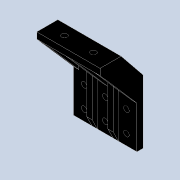
# Autodesk Inventor part: X Axis Drag Chain Support Mount
Saved by Autodesk Inventor 2022 (Build 260153000, 153)
## iProperties
Created: 2021-10-30
Part Number: X Axis Drag Chain Support Mount
Material: Generic
Document SubType Name: Modeling
Designer: Coy
Density: 1 g/cm^3
Appearance: Anodized - Black
Author: Coy
Autodesk Inventor part; units mm, degrees
ref_plane "YZ Plane" through (0, 0, 0) normal (1, 0, 0) x (0, 1, 0)
ref_plane "XZ Plane" through (0, 0, 0) normal (0, 1, 0) x (-1, 0, 0)
sketch "Sketch1" plane through (0, 0, 0) normal (0, 0, 1) x (1, 0, 0)
  line L0 (0, 0) -> (-60, 0)
  line L1 (-60, 0) -> (-60, 60)
  line L2 (-60, 60) -> (0, 60)
  line L3 (0, 60) -> (0, 0)
  dimension "d0" = 60
  dimension "d1" = 60
  constraints: 8 end point, 2 parallel, 1 horizontal, 1 perpendicular
  measures "d0" distance of L1.end L2.end
  measures "d1" distance of L0.end L1.end
extrude "Extrusion1" add sketch "Sketch1" along normal blind 6
sketch "Sketch2" plane through (0, 0, 6) normal (0, 0, 1) x (1, 0, 0)
  line L0 (0, 60) -> (-60, 60) projected
  line L1 (-60, 60) -> (-60, 0) projected
  line L2 (0, 60) -> (-60, 60)
  line L3 (-60, 60) -> (-60, 40)
  line L4 (-60, 40) -> (0, 40)
  line L5 (0, 40) -> (0, 60)
  line L6 (-60, 0) -> (0, 0) construction
  line L7 (-30, 0) -> (-30, 40) construction
  line L8 (-30, 20) -> (-30, 40) construction
  line L9 (-30, 20) -> (-30, 0) construction
  line L10 (-60, 30) -> (0, 30) construction
  line L11 (0, 0) -> (0, 60) construction
  line L12 (-60, 10) -> (0, 10) construction
  circle A0 centre (-50, 30) radius 2.6
  circle A1 centre (-30, 30) radius 2.6
  circle A2 centre (-10, 30) radius 2.6
  circle A3 centre (-50, 10) radius 2.6
  circle A4 centre (-30, 10) radius 2.6
  circle A5 centre (-10, 10) radius 2.6
  dimension "d4" = 20
  dimension "d5" = 5.2
  dimension "d6" = 5.2
  dimension "d7" = 5.2
  dimension "d8" = 5.2
  dimension "d9" = 5.2
  dimension "d10" = 5.2
  dimension "d11" = 20
  dimension "d12" = 20
  dimension "d13" = 20
  dimension "d14" = 20
  dimension "d15" = 20
  constraints: 18 end point, 8 midpoint, 6 centre point, 6 point on line, 2 collinear, 2 parallel, 2 perpendicular, 1 horizontal
  measures "d4" distance of L3.end L2.end
  measures "d5" diameter of A0
  measures "d6" diameter of A1
  measures "d7" diameter of A2
  measures "d8" diameter of A3
  measures "d9" diameter of A4
  measures "d10" diameter of A5
  measures "d11" distance of A1.centre A0.centre
  measures "d12" distance of A4.centre A3.centre
  measures "d13" distance of A1.centre A2.centre
  measures "d14" distance of A4.centre A5.centre
  measures "d15" distance between parallel lines of L10 L12
extrude "Extrusion2" cut sketch "Sketch2" against normal up to next contours A0 | A1 | A2 | A3 | A4 | A5
sketch "Sketch3" plane through (0, 0, 0) normal (1, 0, 0) x (0, 0, -1)
  line L0 (0, 60) -> (0, 0) construction
  line L1 (0, 0) -> (0, 135.0487) construction
  line L2 (-21, 0) -> (-21, 135.0487) construction
  line L3 (-21, 86) -> (-41, 86)
  line L4 (-41, 86) -> (-41, 80)
  line L5 (-41, 80) -> (-21, 80)
  line L6 (-21, 80) -> (-21, 86)
  line L7 (0, 60) -> (-6, 60) projected
  line L8 (0, 60) -> (-6, 60) projected
  line L9 (-21, 86) -> (0, 60)
  line L10 (-6, 60) -> (-6, 0) projected
  line L11 (-6, 60) -> (-21, 80)
  dimension "d18" = 21
  dimension "d19" = 20
  dimension "d20" = 6
  dimension "d21" = 20
  constraints: 16 end point, 2 parallel, 2 vertical, 1 horizontal, 1 perpendicular, 1 point on line
  measures "d18" distance between parallel lines of L1 L2
  measures "d19" distance of L5.end L4.end
  measures "d20" distance of L4.end L3.end
  measures "d21" distance between parallel lines of L7 L5
extrude "Extrusion3" add sketch "Sketch3" against normal up to surface (60 mm away)
sketch "Sketch4" plane through (0, 80, 41) normal (0, 0, 1) x (1, 0, 0)
  line L0 (0, 0) -> (-60, 0) projected
  line L1 (0, 0) -> (-5, 0)
  line L2 (-5, 0) -> (-5, -40)
  line L3 (-5, -40) -> (0, -40)
  line L4 (0, -40) -> (0, 0)
  circle A0 centre (-10, -50) radius 2.6 projected
  line L5 (-32.5, 0) -> (-32.5, -40)
  line L6 (-27.5, 0) -> (-32.5, 0)
  line L7 (-27.5, -40) -> (-27.5, 0)
  line L8 (-32.5, -40) -> (-27.5, -40)
  line L9 (-60, 0) -> (-60, -40)
  line L10 (-55, 0) -> (-60, 0)
  line L11 (-55, -40) -> (-55, 0)
  line L12 (-60, -40) -> (-55, -40)
  point P0 (0, -80)
  dimension "d24" = 5
  dimension "d25" = 10
  dimension "d28" = 27.5
  constraints: 24 end point, 2 horizontal, 2 parallel, 1 perpendicular, 16 other
  measures "d24" distance of L3.end L2.end
  measures "d25" distance from line of A0.centre L3
  measures "d28" distance of L1.end L5.start
extrude "Extrusion4" add sketch "Sketch4" against normal up to next contours L4 L3 L2 L0 | L11 L12 L9 L0 | L7 L8 L5 L0
chamfer "Chamfer1" distance 40 distance2 35 1 edges at (-2.5, 40, 41) measured on face at (-30.8333, 84, 41)
chamfer "Chamfer2" distance 40 distance2 35 1 edges at (-30, 40, 41) measured on face at (-30.8333, 84, 41)
chamfer "Chamfer3" distance 40 distance2 35 1 edges at (-57.5, 40, 41) measured on face at (-30.8333, 84, 41)
sketch "Sketch5" plane through (-55, 80, 21) normal (0, -1, 0) x (1, 0, 0)
  line L0 (-5, 0) -> (-5, 20) construction
  line L1 (-5, 10) -> (55, 10) construction
  line L2 (55, -15) -> (55, 20) construction
  circle A0 centre (11.25, 10) radius 2.6
  circle A1 centre (38.75, 10) radius 2.6
  line L3 (0, 20) -> (0, 0) projected
  line L4 (27.5, 20) -> (27.5, 0) projected
  point P0 (55, -21)
  dimension "d44" = 5.2
  dimension "d45" = 5.2
  dimension "d46" = 11.25
  dimension "d47" = 11.25
  constraints: 3 point on line, 2 centre point, 2 end point, 1 horizontal, 1 midpoint
  measures "d44" diameter of A0
  measures "d45" diameter of A1
  measures "d46" distance from line of L3 A0.centre
  measures "d47" distance from line of L4 A1.centre
extrude "Extrusion5" cut sketch "Sketch5" against normal up to next
ref_plane "Work Plane1" through (0, 0, 11) normal (0, 0, 1) x (1, 0, 0)
sketch "Sketch7" plane through (0, 0, 11) normal (0, 0, 1) x (1, 0, 0)
  line L0 (-60, 0) -> (0, 0) projected
  line L1 (-17.5, 0) -> (-22.5, 0)
  line L2 (-22.5, 0) -> (-22.5, 70)
  line L3 (-22.5, 70) -> (-17.5, 70)
  line L4 (-17.5, 70) -> (-17.5, 0)
  circle A0 centre (-10, 30) radius 2.6 projected
  line L5 (-30, 0) -> (-30, 54.0913) construction
  line L6 (-42.5, 0) -> (-37.5, 0)
  line L7 (-37.5, 0) -> (-37.5, 70)
  line L8 (-37.5, 70) -> (-42.5, 70)
  line L9 (-42.5, 70) -> (-42.5, 0)
  dimension "d68" = 5
  dimension "d69" = 70
  dimension "d70" = 7.5
  constraints: 18 end point, 4 symmetric about line, 2 parallel, 1 horizontal, 1 midpoint, 1 perpendicular, 1 point on line, 1 vertical
  measures "d68" distance of L2.end L3.end
  measures "d69" distance of L1.end L2.end
  measures "d70" distance from line of A0.centre L4
extrude "Extrusion7" add sketch "Sketch7" against normal up to next contours L9 L8 L7 L0 | L2 L3 L4 L0
chamfer "Chamfer8" distance 10 distance2 5 1 edges at (-20, 0, 11) measured on face at (-19.1667, 22.2222, 11)
chamfer "Chamfer9" distance 10 distance2 5 1 edges at (-40, 0, 11) measured on face at (-39.1667, 22.2222, 11)
chamfer "Chamfer10" distance 16.6667 distance2 10 1 edges at (-40, 66.6667, 11) measured on face at (-43.3333, 75.5556, 17.6667)
chamfer "Chamfer11" distance 16.6667 distance2 10 1 edges at (-20, 66.6667, 11) measured on face at (-16.6667, 75.5556, 17.6667)
equation "\"d6\" = d5"
equation "\"d7\" = d5"
equation "\"d8\" = d5"
equation "\"d9\" = d5"
equation "\"d10\" = d5"
equation "\"d47\" = d46"
body "Solid1"
